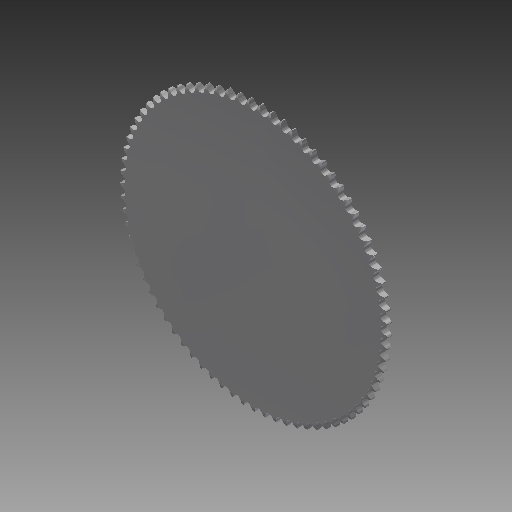
# Autodesk Inventor part: Roller Chain Sprocket2
Saved by Autodesk Inventor 2017 (Build 210142000, 142)
## iProperties
Created: 2016-10-04
Part Number: Roller Chain Sprocket2
Material: Steel
Document SubType Name: Modeling
Designer: hanso
Density: 1 g/cm^3
Appearance: Steel
CustomPartVersion: 1
Author: hanso
Autodesk Inventor part; units mm, degrees
ref_plane "YZ Plane" through (0, 0, 0) normal (1, 0, 0) x (0, 1, 0)
ref_plane "XZ Plane" through (0, 0, 0) normal (0, 1, 0) x (-1, 0, 0)
sketch "Theoretical Tooth Profile" plane through (0, 0, 0) normal (0, 0, 1) x (1, 0, 0)
  circle A0 centre (0, 0) radius 155.6808 construction
  line L0 (0, 0) -> (0, 155.6808) construction
  line L1 (0, 0) -> (12.6894, 155.1628) construction
  circle A1 centre (0, 0) radius 159.3612
  arc A2 (-3.2616, 153.3303) -> (3.2616, 153.3303) centre (0, 155.6808) ccw
  line L2 (0, 155.6808) -> (12.6894, 155.1628) construction
  line L3 (0, 155.6808) -> (5.1434, 159.3875) construction
  line L4 (5.1434, 159.3875) -> (-4.681, 156.099) construction
  arc A3 (6.1653, 159.2419) -> (5.0642, 157.2437) centre (11.0855, 155.2283) ccw
  arc A4 (-5.0642, 157.2437) -> (-6.1653, 159.2419) centre (-11.0855, 155.2283) ccw
  line L5 (-11.0855, 155.2283) -> (-5.0642, 157.2437) construction
  arc A5 (-4.681, 156.099) -> (-3.2616, 153.3303) centre (5.1434, 159.3875) ccw
  line L6 (-4.681, 156.099) -> (-5.0642, 157.2437)
  arc A6 (3.2616, 153.3303) -> (4.681, 156.099) centre (-5.1434, 159.3875) ccw
  line L7 (5.0642, 157.2437) -> (4.681, 156.099)
  line L8 (0, 0) -> (6.5001, 159.2286) construction
  point P0 (6.3447, 155.4218)
  dimension "d0" = 311.3616
  dimension "d2" = 4.675
  dimension "d3" = 4.0203
  dimension "d10" = 125.779
  dimension "d11" = 17.273
  dimension "d12" = 6.3398
  dimension "d13" = 10.3602
  dimension "d14" = 11.0947
  dimension "d23" = 3.81
  constraints: 18 end point, 15 point on circle, 7 centre point, 3 coincident, 3 point on line, 3 symmetric about line, 3 tangent, 1 equal radius, 1 midpoint, 1 parallel, 1 vertical, 1 other
  measures "d0" diameter of A0
  measures "d2" angle of L1 L0
  measures "d3" radius of A2
  measures "d10" angle of L3 L0
  measures "d11" angle of L4 L3
  measures "d12" distance of L2.start L3.end
  measures "d13" distance of L3.end L4.end
  measures "d14" distance of A3.centre L0.end
  measures "d23" distance from line of L8.end L2
sketch "Tooth Profile" plane through (0, 0, 0) normal (0, 0, 1) x (1, 0, 0)
  circle A0 centre (0, 0) radius 159.3612 projected
  line L0 (0, 0) -> (0, 155.6808) construction
  line L1 (0, 155.6808) -> (3.7636, 154.2673) construction
  arc A1 (-3.7636, 154.2673) -> (3.7636, 154.2673) centre (0, 155.6808) ccw
  line L2 (-3.7636, 154.2673) -> (0, 155.6808) construction
  arc A2 (-3.7636, 154.2673) -> (-5.844, 159.2541) centre (-74.0943, 127.8536) ccw
  arc A3 (5.844, 159.2541) -> (3.7636, 154.2673) centre (74.0943, 127.8536) ccw
  dimension "d44" = 138.831
  dimension "d45" = 4.0203
  dimension "d46" = 75.1271
  constraints: 8 point on circle, 7 end point, 3 centre point, 2 tangent, 1 coincident, 1 equal radius, 1 symmetric about line, 1 vertical
  measures "d44" angle of L1 L2
  measures "d45" radius of A1
  measures "d46" radius of A3
sketch "Section Profile" plane through (0, 0, 0) normal (1, 0, 0) x (0, 1, 0)
  line L0 (159.3612, 0) -> (-159.3612, 0) projected
  line L1 (148.3122, 3.7612) -> (-148.3122, 3.7612)
  line L2 (-148.3122, 3.7612) -> (-148.3122, -3.7612)
  line L3 (-148.3122, -3.7612) -> (148.3122, -3.7612)
  line L4 (148.3122, -3.7612) -> (148.3122, 3.7612)
  line L5 (148.3122, 3.7612) -> (159.3612, 3.7612) construction
  line L6 (159.3612, 3.7612) -> (159.3612, -3.7612) construction
  line L7 (159.3612, -3.7612) -> (148.3122, -3.7612) construction
  line L8 (148.3122, -3.7612) -> (148.3122, 3.7612)
  arc A0 (159.3612, 2.1737) -> (153.0097, 3.7612) centre (153.0097, -9.7389) ccw
  arc A1 (153.0097, -3.7612) -> (159.3612, -2.1737) centre (153.0097, 9.7389) ccw
  line L9 (153.0097, 3.7612) -> (0, 3.7612)
  line L10 (0, 3.7612) -> (0, -3.7612)
  line L11 (0, -3.7612) -> (153.0097, -3.7612)
  line L12 (0, 3.7612) -> (0, -3.7612)
  line L13 (159.3612, 2.1737) -> (159.3612, -2.1737)
  point P0 (0, 0)
  point P1 (0, 0)
  dimension "d30" = 7.5225
  dimension "d31" = 296.6245
  dimension "d32" = 7.5225
  dimension "d33" = 1.5875
  dimension "d34" = 13.5001
  dimension "d43" = 3.7612
  constraints: 26 end point, 7 midpoint, 5 perpendicular, 4 parallel, 4 point on circle, 3 point on line, 3 symmetric about line, 2 centre point, 2 horizontal, 2 tangent, 1 collinear, 1 other
  measures "d30" distance between parallel lines of L7 L5
  measures "d31" distance between parallel lines of L2 L4
  measures "d32" distance between parallel lines of L3 L1
  measures "d33" distance from line of L13.start L5
  measures "d34" radius of A0
  measures "d43" distance between parallel lines of L3 L0
revolve "Shroud" add sketch "Section Profile" angle 360 about axis through (0, 0, 3.7612) along (0, 0, -1) contours L10 L3 L2 L0 | L0 L2 L1 L10
revolve "Strand" add sketch "Section Profile" angle 360 about axis through (0, 0, 3.7612) along (0, 0, -1) contours L13 A1 L11 L4 L0 | L0 L4 L9 A0 L13 | L4 L3 L10 L0 | L0 L10 L1 L4
pattern_of_one "Strand Pattern"
extrude "Theoretical Tooth" cut sketch "Theoretical Tooth Profile" along normal through all both and the other way through all contours A3 L7 A6 A2 A5 L6 A4 A1 picked at (0.6852, 155.3362)
extrude "Tooth" [suppressed]
pattern_circular "Tooth Pattern" count 77 over 360 about axis through (0, 0, -10) along (0, 0, 1) of "Theoretical Tooth"
ref_plane "Timing Plane" through (0, 155.6808, 0) normal (1, 0, 0) x (0, 1, 0)
equation "\"d3\" = 0.5 * da_Dr + da_SC"
equation "\"d12\" = 0.8 * da_Dr"
equation "\"d13\" = 1.3 * da_Dr + da_SC"
equation "\"d14\" = 1.4 * da_Dr"
equation "\"d23\" = da_Ha"
equation "\"d44\" = da_Alfa"
equation "\"d45\" = da_Ri"
equation "\"d46\" = da_Re"
equation "\"d30\" = da_Bf"
equation "\"d31\" = da_Ds"
equation "\"d32\" = da_Bs"
equation "\"d33\" = da_Ba"
equation "\"d34\" = da_Rx"
equation "\"d40\" = da_pt"
equation "\"form_type\" = 0"
equation "\"da_p\" = 12.7"
equation "\"da_Dr\" = 7.9248"
equation "\"da_SC\" = 0.05791"
equation "\"da_Ha\" = 3.81"
equation "\"da_pt\" = 14.3764"
equation "\"da_Bf\" = 7.52246"
equation "\"da_Ba\" = 1.5875"
equation "\"da_Rx\" = 13.5001"
equation "\"da_Ra\" = 0.508"
equation "\"da_Bs\" = 7.52246"
equation "\"da_Ds\" = 296.6245"
equation "\"da_Re\" = 75.1271"
equation "\"da_Ri\" = 4.02031"
equation "\"da_Alfa\" = 138.831deg"
body "Solid1"
